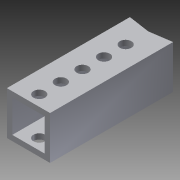
# Autodesk Inventor part: V mount
Saved by Autodesk Inventor 2013 (Build 170138000, 138)
## iProperties
Created: 2013-02-04
Part Number: V mount
Material: Aluminum 6061
Document SubType Name: Modeling
Designer: Arpan
Density: 1 g/cm^3
Author: Arpan
Autodesk Inventor part; units mm, degrees
ref_plane "YZ Plane" through (0, 0, 0) normal (1, 0, 0) x (0, 1, 0)
ref_plane "XZ Plane" through (0, 0, 0) normal (0, 1, 0) x (-1, 0, 0)
ref_plane "XY Plane" through (0, 0, 0) normal (0, 0, 1) x (1, 0, 0)
sketch "Sketch1" plane through (0, 0, 0) normal (0, 0, 1) x (1, 0, 0)
  line L0 (0, 0) -> (-25.4, 0)
  line L1 (-25.4, 0) -> (-25.4, 25.4)
  line L2 (-25.4, 25.4) -> (0, 25.4)
  line L3 (0, 25.4) -> (0, 0)
  line L4 (-3.175, 22.225) -> (-22.225, 22.225)
  line L5 (-22.225, 22.225) -> (-22.225, 3.175)
  line L6 (-22.225, 3.175) -> (-3.175, 3.175)
  line L7 (-3.175, 3.175) -> (-3.175, 22.225)
  dimension "d2" = 25.4
  dimension "d4" = 25.4
  dimension "d5" = 3.175
  constraints: 16 end point, 4 parallel, 2 perpendicular, 1 horizontal, 3 other
  measures "d2" distance of L0.end L1.end
  measures "d4" distance of L1.end L2.end
  measures "d5" distance between parallel lines of L2 L4
extrude "Extrusion1" add sketch "Sketch1" along normal blind 72.39
sketch "Sketch2" plane through (-25.4, 25.4, 0) normal (0, 1, 0) x (1, 0, 0)
  line L0 (0, 0) -> (25.4, 0) projected
  line L1 (0, 0) -> (0, -72.39) projected
  line L2 (0, 0) -> (0, -1.905)
  line L3 (12.7, 0) -> (12.7, -1.905)
  line L4 (12.7, -1.905) -> (0, 0)
  line L5 (12.7, -1.905) -> (25.4, 0)
  dimension "d8" = 1.905
  dimension "d9" = 1.905
  constraints: 8 end point, 1 midpoint, 1 parallel, 1 point on line
  measures "d8" distance of L0.start L2.end
  measures "d9" distance of L3.start L3.end
extrude "Extrusion2" cut sketch "Sketch2" against normal blind 25.4
sketch "Sketch3" plane through (-25.4, 25.4, 72.39) normal (0, 1, 0) x (1, 0, 0)
  line L0 (25.4, 0) -> (0, 0) projected
  line L1 (25.4, 72.39) -> (25.4, 0) projected
  line L2 (12.7, 0) -> (12.7, 70.485) construction
  line L3 (12.7, 0) -> (12.7, 6.35)
  circle A0 centre (12.7, 6.35) radius 3.3782
  circle A1 centre (12.7, 19.05) radius 3.3782
  circle A2 centre (12.7, 31.75) radius 3.3782
  circle A3 centre (12.7, 44.45) radius 3.3782
  circle A4 centre (12.7, 57.15) radius 3.3782
  dimension "d12" = 6.35
  dimension "d13" = 6.7564
  dimension "d16" = 12.7
  constraints: 5 centre point, 4 end point, 1 coincident, 1 midpoint, 1 parallel, 1 point on line, 1 vertical, 8 other
  measures "d12" distance of L2.start L3.end
  measures "d13" diameter of A0
  measures "d16" distance of A0.centre A1.centre
extrude "Extrusion3" cut sketch "Sketch3" against normal blind 25.4
body "Solid1"
